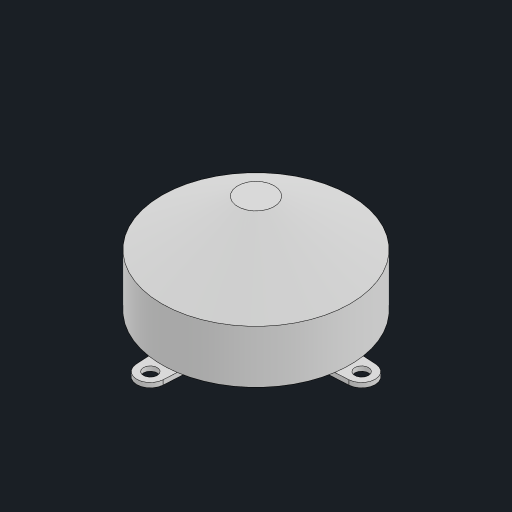
# Autodesk Inventor part: MainMotor._Newipt
Saved by Autodesk Inventor 2023 (Build 270158000, 158)
## iProperties
Created: 2022-07-26
Part Number: MainMotor._Newipt
Material: 一般
Document SubType Name: Modeling
Designer: legot
Density: 1 g/cm^3
Appearance: 既定
Author: legot
Autodesk Inventor part; units mm, degrees
ref_plane "YZ Plane" through (0, 0, 0) normal (1, 0, 0) x (0, 1, 0)
ref_plane "XZ Plane" through (0, 0, 0) normal (0, 1, 0) x (-1, 0, 0)
ref_plane "XY Plane" through (0, 0, 0) normal (0, 0, 1) x (1, 0, 0)
sketch "スケッチ1" plane through (0, 0, 0) normal (1, 0, 0) x (0, 1, 0)
  line L0 (0, 0) -> (15, 0)
  line L1 (15, 0) -> (15, -2.75)
  line L2 (15, -2.75) -> (8, -14.25)
  line L3 (8, -14.25) -> (0, -14.25)
  line L4 (0, -14.25) -> (0, 0)
  dimension "d0" = 14.25
  dimension "d1" = 15
  dimension "d2" = 2.75
  dimension "d3" = 8
  constraints: 10 end point, 2 perpendicular, 1 horizontal, 1 parallel
  measures "d0" distance of L3.end L0.start
  measures "d1" distance of L0.start L0.end
  measures "d2" distance of L0.end L1.end
  measures "d3" distance of L2.end L3.end
revolve "回転1" add sketch "スケッチ1" angle 360 about axis through (0, 0, 0) along (0, 1, 0)
sketch "スケッチ2" plane through (0, 0, 0) normal (0, -1, 0) x (1, 0, 0)
  circle A0 centre (0, 16) radius 1.05
  circle A1 centre (0, 8) radius 1.5
  arc A2 (2.0468, 16.1153) -> (-2.0468, 16.1153) centre (0, 16) ccw
  line L0 (2.0468, 16.1153) -> (2.5458, 7.2567)
  line L1 (-2.0468, 16.1153) -> (-2.5458, 7.2567)
  circle A3 centre (0, 0) radius 14.25 construction
  circle A4 centre (0, 8) radius 2.5 construction
  arc A5 (2.5458, 7.2567) -> (7.2567, 2.5458) centre (7.5379, 7.5379) ccw
  circle A6 centre (-16, 0) radius 1.05
  circle A7 centre (-8, 0) radius 1.5
  arc A8 (-16.1153, 2.0468) -> (-16.1153, -2.0468) centre (-16, 0) ccw
  line L2 (-16.1153, 2.0468) -> (-7.2567, 2.5458)
  line L3 (-16.1153, -2.0468) -> (-7.2567, -2.5458)
  circle A9 centre (-8, 0) radius 2.5 construction
  arc A10 (-7.2567, 2.5458) -> (-2.5458, 7.2567) centre (-7.5379, 7.5379) ccw
  circle A11 centre (0, -16) radius 1.05
  circle A12 centre (0, -8) radius 1.5
  arc A13 (-2.0468, -16.1153) -> (2.0468, -16.1153) centre (0, -16) ccw
  line L4 (-2.0468, -16.1153) -> (-2.5458, -7.2567)
  line L5 (2.0468, -16.1153) -> (2.5458, -7.2567)
  circle A14 centre (0, -8) radius 2.5 construction
  arc A15 (-2.5458, -7.2567) -> (-7.2567, -2.5458) centre (-7.5379, -7.5379) ccw
  circle A16 centre (16, 0) radius 1.05
  circle A17 centre (8, 0) radius 1.5
  arc A18 (16.1153, -2.0468) -> (16.1153, 2.0468) centre (16, 0) ccw
  line L6 (16.1153, -2.0468) -> (7.2567, -2.5458)
  line L7 (16.1153, 2.0468) -> (7.2567, 2.5458)
  circle A19 centre (8, 0) radius 2.5 construction
  arc A20 (7.2567, -2.5458) -> (2.5458, -7.2567) centre (7.5379, -7.5379) ccw
  point P0 (7.2567, 2.5458)
  dimension "d5" = 2.1
  dimension "d6" = 3
  dimension "d7" = 16
  dimension "d8" = 1
  dimension "d9" = 1
  dimension "d10" = 5
  dimension "d13" = 360
  dimension "d15" = 8
  constraints: 20 centre point, 16 end point, 16 point on circle, 5 tangent, 2 vertical alignment, 1 coincident, 1 equal length, 61 other
  measures "d5" diameter of A0
  measures "d6" diameter of A1
  measures "d7" distance of A0.centre A3.centre
  measures "d8" radial gap between concentric circles of A0 A2
  measures "d9" radial gap between concentric circles of A1 A4
  measures "d10" radius of A5
  measures "d15" distance of A1.centre A3.centre
extrude "押し出し1" add sketch "スケッチ2" along normal blind 0.7
